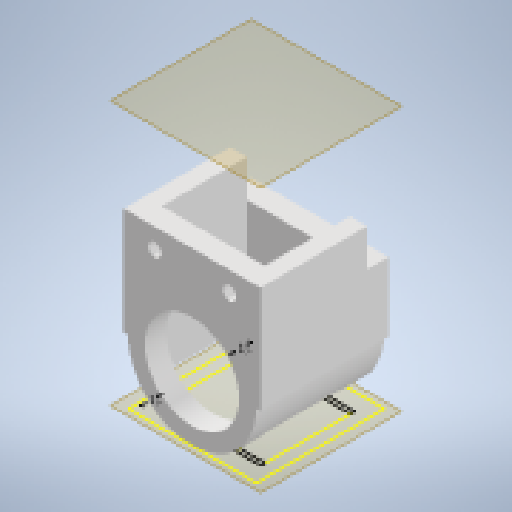
# Autodesk Inventor part: arm1
Saved by Autodesk Inventor 2024 (Build 280153000, 153)
## iProperties
Created: 2025-11-24
Part Number: arm1
Material: Generic
Document SubType Name: Modeling
Designer: Aidan
Density: 1 g/cm^3
Appearance: Default
Author: Aidan
Autodesk Inventor part; units mm, degrees
ref_plane "YZ Plane" through (0, 0, 0) normal (1, 0, 0) x (0, 1, 0)
ref_plane "XY Plane" through (0, 0, 0) normal (0, 0, 1) x (1, 0, 0)
sketch "Sketch1" plane through (0, 0, 0) normal (0, 0, 1) x (1, 0, 0)
  line L0 (-17.25, -31.85) -> (4.85, -31.85) projected
  line L1 (4.85, -31.85) -> (4.85, 0) projected
  arc A0 (4.85, 0) -> (0, 4.85) centre (0, 0) ccw projected
  line L2 (0, 4.85) -> (-12.4, 4.85) projected
  arc A1 (-12.4, 4.85) -> (-17.25, 0) centre (-12.4, 0) ccw projected
  line L3 (-17.25, 0) -> (-17.25, -31.85) projected
  circle A2 centre (-6.2, -6.5) radius 2.75 projected
  circle A3 centre (-6.2, -17.15) radius 1.95 projected
  arc A4 (1.9991, -27.9755) -> (1.0928, -27.0978) centre (2.55, -26.5) ccw projected
  arc A5 (1.0928, -27.0978) -> (1.9991, -27.9755) centre (-0.065, -29.2) ccw projected
  arc A6 (-13.4928, -27.0978) -> (-14.3991, -27.9755) centre (-14.95, -26.5) ccw projected
  arc A7 (-14.3991, -27.9755) -> (-13.4928, -27.0978) centre (-12.335, -29.2) ccw projected
  line L4 (9.85, -61.85) -> (-22.25, -61.85)
  line L5 (-22.25, -61.85) -> (-22.25, -21.85)
  line L6 (-22.25, -21.85) -> (9.85, -21.85)
  line L7 (9.85, -21.85) -> (9.85, -61.85)
  circle A8 centre (2.55, -26.5) radius 1.575
  circle A9 centre (-14.95, -26.5) radius 1.575
  point P0 (0, 0)
  point P1 (1.0928, -27.0978)
  point P2 (1.9991, -27.9755)
  point P3 (-17.25, -21.85)
  point P4 (4.85, -21.85)
  dimension "d2" = 5
  dimension "d3" = 5
  dimension "d12" = 10
  dimension "d13" = 40
  constraints: 8 end point, 2 centre point, 2 coincident, 2 concentric, 2 parallel, 1 horizontal, 1 perpendicular
  measures "d2" distance between parallel lines of L3 L5
  measures "d3" distance between parallel lines of L7 L1
  measures "d12" distance between parallel lines of L6 L0
  measures "d13" distance of L6.end L4.start
extrude "Extrusion2" add sketch "Sketch1" along normal blind 5 contours L3 L6 L1 L0 | L0 L1 L6 L7 L4 L5 L3 | A5 A8 | A7 A9
sketch "Sketch2" plane through (0, 0, 0) normal (0, 0, -1) x (-1, 0, 0)
  line L0 (22.25, -21.85) -> (22.25, -61.85) projected
  line L1 (22.25, -61.85) -> (18.25, -61.85)
  line L2 (18.25, -61.85) -> (18.25, -21.85)
  line L3 (18.25, -21.85) -> (22.25, -21.85)
  line L4 (22.25, -21.85) -> (22.25, -61.85)
  line L5 (-9.85, -61.85) -> (-9.85, -21.85) projected
  line L6 (-9.85, -21.85) -> (22.25, -21.85) projected
  line L7 (-9.85, -61.85) -> (-5.85, -61.85)
  line L8 (-5.85, -61.85) -> (-5.85, -21.85)
  line L9 (-5.85, -21.85) -> (-9.85, -21.85)
  line L10 (-9.85, -21.85) -> (-9.85, -61.85)
  point P0 (0, 0)
  point P1 (-4.85, -21.85)
  point P2 (17.25, -21.85)
  point P3 (-9.85, -21.85)
  dimension "d8" = 4
  dimension "d9" = 4
  constraints: 16 end point, 4 parallel, 2 horizontal, 2 perpendicular, 1 collinear, 1 point on line
  measures "d8" distance of L2.end L3.end
  measures "d9" distance of L9.end L8.end
extrude "Extrusion3" add sketch "Sketch2" along normal blind 20
sketch "Sketch3" plane through (0, 0, -20) normal (0, 0, -1) x (-1, 0, 0)
  circle A0 centre (-2.55, -26.5) radius 1.575 projected
  circle A1 centre (14.95, -26.5) radius 1.575 projected
  circle A2 centre (6.2, -6.5) radius 2.95 projected
  line L0 (-43.9339, 5.041) -> (56.0661, 5.041) projected
  line L1 (-23.9339, -29.6) -> (-43.9339, 5.041) projected
  line L2 (36.0661, -29.6) -> (-23.9339, -29.6) projected
  line L3 (56.0661, 5.041) -> (36.0661, -29.6) projected
  line L4 (22.25, -61.85) -> (-9.85, -61.85) projected
  line L5 (-9.85, -61.85) -> (-9.85, -21.85) projected
  line L6 (22.25, -61.85) -> (-9.85, -61.85)
  line L7 (-9.85, -61.85) -> (-9.85, -30.6)
  line L8 (-9.85, -30.6) -> (22.25, -30.6)
  line L9 (22.25, -30.6) -> (22.25, -61.85)
  point P0 (0, 0)
  dimension "d14" = 1
  constraints: 8 end point, 2 parallel, 1 horizontal, 1 perpendicular, 1 point on line
  measures "d14" distance between parallel lines of L8 L2
extrude "Extrusion4" add sketch "Sketch3" along normal blind 5 contours L8 L9 L4 L5
sketch "Sketch4" plane through (0, 0, 5) normal (0, 0, 1) x (1, 0, 0)
  circle A0 centre (-6.2, -46.85) radius 11.05
  line L0 (-22.25, -21.85) -> (-22.25, -61.85) projected
  line L1 (-22.25, -61.85) -> (9.85, -61.85) projected
  point P0 (0, 0)
  dimension "d17" = 22.1
  dimension "d18" = 16.05
  dimension "d19" = 15
  constraints: 1 centre point
  measures "d17" diameter of A0
  measures "d18" distance from line of L0 A0.centre
  measures "d19" distance from line of L1 A0.centre
extrude "Extrusion5" cut sketch "Sketch4" against normal up to surface (5 mm away)
sketch "Sketch5" plane through (0, 0, -25) normal (0, 0, -1) x (-1, 0, 0)
  circle A0 centre (6.2, -46.85) radius 4.508
  circle A1 centre (6.2, -46.85) radius 15
  line L0 (22.25, -21.85) -> (22.25, -61.85) projected
  line L1 (22.25, -46.85) -> (-9.85, -46.85)
  line L2 (-9.85, -61.85) -> (-9.85, -21.85) projected
  line L3 (22.25, -46.85) -> (22.25, -61.85)
  line L4 (22.25, -61.85) -> (-9.85, -61.85)
  line L5 (-9.85, -46.85) -> (-9.85, -61.85)
  point P0 (0, 0)
  point P1 (6.2, -61.85)
  point P2 (21.2, -46.85)
  point P3 (-8.8, -46.85)
  dimension "d22" = 30
  constraints: 8 end point, 2 centre point, 2 collinear, 2 point on line, 1 coincident, 1 horizontal, 1 midpoint, 1 perpendicular, 2 other
  measures "d22" diameter of A1
extrude "Extrusion6" cut sketch "Sketch5" against normal up to surface (30 mm away) contours L1 L0 L4 A1 | A1 L4 L2 L1
ref_plane "Work Plane1" through (-6.2, -61.85, -25) normal (0, 1, 0) x (-1, 0, 0)
sketch "Sketch6" plane through (-6.2, -61.85, -25) normal (0, 1, 0) x (-1, 0, 0)
  line L0 (-15, 0) -> (15, 0) projected
  line L1 (-15, 0) -> (-15, 30) projected
  line L2 (15, 30) -> (-15, 30) projected
  line L3 (15, 0) -> (15, 30) projected
  line L4 (12.05, 5) -> (-12.05, 5) projected
  line L5 (12.05, 25) -> (12.05, 5) projected
  line L6 (-12.05, 25) -> (12.05, 25) projected
  line L7 (-12.05, 5) -> (-12.05, 25) projected
  line L8 (-12.05, 25) -> (12.05, 25)
  line L9 (12.05, 25) -> (12.05, 26.5)
  line L10 (12.05, 26.5) -> (-12.05, 26.5)
  line L11 (-12.05, 26.5) -> (-12.05, 25)
  line L12 (-12.05, 5) -> (12.05, 5)
  line L13 (12.05, 5) -> (12.05, 3.5)
  line L14 (12.05, 3.5) -> (-12.05, 3.5)
  line L15 (-12.05, 3.5) -> (-12.05, 5)
  point P0 (-6.2, 25)
  dimension "d25" = 1.5
  dimension "d26" = 1.5
  constraints: 16 end point, 4 parallel, 2 horizontal, 2 perpendicular, 1 collinear, 1 point on line
  measures "d25" distance of L9.end L8.end
  measures "d26" distance of L12.end L13.end
extrude "Extrusion7" cut sketch "Sketch6" along normal up to surface (40 mm away) contours L13 L14 L15 L4 | L6 L11 L10 L9
body "Solid2"
